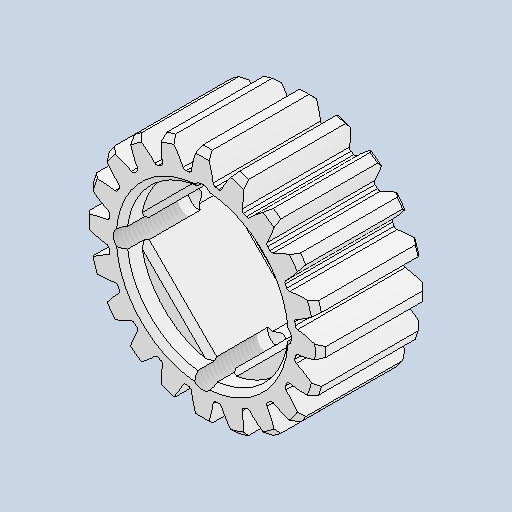
# Autodesk Inventor part: 스퍼 기어1
Saved by Autodesk Inventor 2025.3 (Build 293356030, 356C)
## iProperties
Created: 2025-10-17
Part Number: 스퍼 기어1
Material: PLA filament
Document SubType Name: Modeling
Designer: MSI
Categories: <?xml version="1.0" encoding="UTF-16"?> <MemberInstance><Categories><FamilyTemplate><FamilyTemplateParameter ValueType="xs:double" Id="1" ObjectReferenceKey="da_z" ObjectType="kUserParameterObject"/><FamilyTemplateParameter ValueType="xs:double" Id="2" ObjectReferenceKey="da_b" ObjectType="kUserParameterObject"/><FamilyTemplateParameter ValueType="xs:double" Id="3" ObjectReferenceKey="da_beta" ObjectType="kUserParameterObject"/><FamilyTemplateParameter ValueType="xs:double" Id="4" ObjectReferenceKey="da_da" ObjectType="kUserParameterObject"/><FamilyTemplateParameter ValueType="xs:double" Id="5" ObjectReferenceKey="da_aw" ObjectType="kUserParameterObject"/><FamilyTemplateParameter ValueType="xs:string" Id="6" ObjectReferenceKey="EAIAABAAAACIAQAAAAAAAIAAAAAAAAAA" ObjectType="83910656" SubObjectId="SurfaceGeometry"/></FamilyTemplate><ParamToTemplateMap><ParamToTemplate CategoryParameter="//CategoryParameter[@InternalName='046C89C9-8512-4d59-83FE-43B91F4F132A']" TemplateParameter="1"/><ParamToTemplate CategoryParameter="//CategoryParameter[@InternalName='2552DF32-E462-4b46-AEBF-C6C7768E72AC']" TemplateParameter="2"/><ParamToTemplate CategoryParameter="//CategoryParameter[@InternalName='C9EE641D-15FC-4fae-A226-E94C4372FDD7']" TemplateParameter="3"/><ParamToTemplate><ParamToTemplate CategoryParameter="//CategoryParameter[@InternalName='00B6519A-459B-49c7-AD84-2E56D39A5744']" ConstantValue="0.000000"/></ParamToTemplate><ParamToTemplate><ParamToTemplate CategoryParameter="//CategoryParameter[@InternalName='04B31F0E-C7A6-4894-AA32-9629BEFACF47']" ConstantValue="1.000000"/></ParamToTemplate><ParamToTemplate><ParamToTemplate CategoryParameter="//CategoryParameter[@InternalName='43CBEC2E-7847-49e7-A936-2F7889FCB2D9']" ConstantValue="0.250000"/></ParamToTemplate><ParamToTemplate><ParamToTemplate CategoryParameter="//CategoryParameter[@InternalName='B1EFC894-105D-4ebd-86BF-FA20ED196853']" ConstantValue="0.350000"/></ParamToTemplate><ParamToTemplate><ParamToTemplate CategoryParameter="//CategoryParameter[@InternalName='51175063-3D10-4879-93E8-6246FE8B403D']" ConstantValue="2060000000.000000"/></ParamToTemplate><ParamToTemplate><ParamToTemplate CategoryParameter="//CategoryParameter[@InternalName='A3A52E27-4454-46a9-B0BD-C932399B70AF']" ConstantValue="0.300000"/></ParamToTemplate><ParamToTemplate><ParamToTemplate CategoryParameter="//CategoryParameter[@InternalName='91B76062-C214-41d9-B1B9-14D2AB99603D']" ConstantValue="0.200000"/></ParamToTemplate><ParamToTemplate><ParamToTemplate CategoryParameter="//CategoryParameter[@InternalName='374E806E-8B8A-4dda-A9AA-1039D6500AD2']" ConstantValue="5.000000"/></ParamToTemplate><ParamToTemplate><ParamToTemplate CategoryParameter="//CategoryParameter[@InternalName='2D373A89-B862-43d6-8D0B-0CBF12AB9F6C']" ConstantValue="0.349066"/></ParamToTemplate><ParamToTemplate CategoryParameter="//CategoryParameter[@InternalName='37777632-D6A2-4fac-9D53-DB8ACD95C989']" TemplateParameter="4"/><ParamToTemplate CategoryParameter="//CategoryParameter[@InternalName='FD1017F1-B727-4f7e-9707-0F86F1FF9423']" TemplateParameter="5"/><ParamToTemplate><ParamToTemplate CategoryParameter="//CategoryParameter[@InternalName='9E1B4470-B2D3-4ff1-B813-535BB4CDF51A']" ConstantValue="3520000.000000"/></ParamToTemplate><ParamToTemplate><ParamToTemplate CategoryParameter="//CategoryParameter[@InternalName='F8452263-BFF6-458c-9FB1-07C4B99E95CD']" ConstantValue="11400000.000000"/></ParamToTemplate><ParamToTemplate><ParamToTemplate CategoryParameter="//CategoryParameter[@InternalName='3E3BB259-FD49-497f-8171-6EBC954A3479']" ConstantValue="2.000000"/></ParamToTemplate><ParamToTemplate CategoryParameter="//CategoryParameter[@InternalName='27C3BAF2-7550-4e4b-AE2C-0DB134B7D9B7']" TemplateParameter="6"/></ParamToTemplateMap><Category DisplayName="Gear" InternalName="DC85795E-93AB-48d5-8EEE-5A27447B64BD" Mnemonic="Gear"><CategoryParameter DisplayName="z" InternalName="046C89C9-8512-4d59-83FE-43B91F4F132A" Mnemonic="z"/><CategoryParameter DisplayName="b" InternalName="2552DF32-E462-4b46-AEBF-C6C7768E72AC" Mnemonic="b"/><CategoryParameter DisplayName="||b|" InternalName="C9EE641D-15FC-4fae-A226-E94C4372FDD7" Mnemonic="beta"/><CategoryParameter DisplayName="x" InternalName="00B6519A-459B-49c7-AD84-2E56D39A5744" Mnemonic="x"/><CategoryParameter DisplayName="a*" InternalName="04B31F0E-C7A6-4894-AA32-9629BEFACF47" Mnemonic="a"/><CategoryParameter DisplayName="c*" InternalName="43CBEC2E-7847-49e7-A936-2F7889FCB2D9" Mnemonic="c"/><CategoryParameter DisplayName="r|.f|*" InternalName="B1EFC894-105D-4ebd-86BF-FA20ED196853" Mnemonic="rf"/><CategoryParameter DisplayName="E" InternalName="51175063-3D10-4879-93E8-6246FE8B403D" Mnemonic="E"/><CategoryParameter DisplayName="||m|" InternalName="A3A52E27-4454-46a9-B0BD-C932399B70AF" Mnemonic="mi"/><Category DisplayName="SpurGear" InternalName="26C5A22E-A91E-4dfd-A3B3-23CCAFAE1764" Mnemonic="SpurGear"><CategoryParameter DisplayName="m" InternalName="91B76062-C214-41d9-B1B9-14D2AB99603D" Mnemonic="m"/><CategoryParameter DisplayName="P" InternalName="374E806E-8B8A-4dda-A9AA-1039D6500AD2" Mnemonic="PP"/><CategoryParameter DisplayName="||a|" InternalName="2D373A89-B862-43d6-8D0B-0CBF12AB9F6C" Mnemonic="alpha"/><CategoryParameter DisplayName="d|.a|" InternalName="37777632-D6A2-4fac-9D53-DB8ACD95C989" Mnemonic="da"/><CategoryParameter DisplayName="a|.w|" InternalName="FD1017F1-B727-4f7e-9707-0F86F1FF9423" Mnemonic="aw"/><CategoryParameter DisplayName="||s||.Flim|" InternalName="9E1B4470-B2D3-4ff1-B813-535BB4CDF51A" Mnemonic="sFlim"/><CategoryParameter DisplayName="||s||.Hlim|" InternalName="F8452263-BFF6-458c-9FB1-07C4B99E95CD" Mnemonic="sHlim"/><CategoryParameter DisplayName="유형" InternalName="3E3BB259-FD49-497f-8171-6EBC954A3479" Mnemonic="type"/><CategoryParameter DisplayName="PitchDiameter" InternalName="27C3BAF2-7550-4e4b-AE2C-0DB134B7D9B7" Mnemonic="IDS_PITCHDIAM"/></Category></Category></Categories></MemberInstance>
Density: 1.2 g/cm^3
Appearance: 일반
Mass: 16.1847 g
Surface Area: 81.0229 cm^2
Volume: 13.4873 cm^3
Author: MSI
Autodesk Inventor part; units mm, degrees
sketch "Sketch1" plane through (0, 0, 0) normal (0, 0, 1) x (1, 0, 0)
  circle A0 centre (0, 0) radius 22
  dimension "d0" = 44
  constraints: 1 centre point
  measures "d0" diameter of A0
extrude "Extrusion1" add sketch "Sketch1" along normal blind 20
chamfer "모따기1" distance 1 angle 45 2 edges at (-22, 0, 0) (-22, 0, 20)
ref_plane "Work Plane2" through (0, 0, 10) normal (0, 0, 1) x (1, 0, 0)
sketch "Sketch2" plane through (0, 0, 0) normal (0, 0, -1) x (-1, 0, 0)
  circle A0 centre (0, 0) radius 22 projected
  circle A1 centre (0, 0) radius 20
  dimension "d3" = 40
  constraints: 1 centre point, 1 coincident
  measures "d3" diameter of A1
surface extrude "피치 지름" sketch "Sketch2" against normal through all shown no curves A1
ref_plane "Work Plane8" through (0, 0, 0) normal (0.9876883, 0.1564345, 0) x (0, 0, 1)
ref_plane "Work Plane9" through (0, 0, 0) normal (1, 0, 0) x (0, 1, 0)
spur gear teeth "스퍼 기어" teeth 20 pitch diameter 40 tip diameter 44 root diameter 35 face width 20 start plane through (0, 0, 0) normal (0, 0, -1) x (-1, 0, 0)
fillet "모깎기1" radius 0.5 2 edges at (2.0569, 17.3787, 10) (3.4141, 17.1637, 10)
pattern_circular "원형 패턴1" count 20 over 360 about axis through (0, 0, 0) along (0, 0, 1) of "모깎기1"
sketch "스케치3" plane through (0, 0, 20) normal (0, 0, 1) x (1, 0, 0)
  point P0 (0, 0)
hole "구멍1" at (0, 0, 20) direction (0, 0, -1) diameter 30 end through all
sketch "스케치5" plane through (0, 0, 0) normal (0, 0, 1) x (1, 0, 0)
  line L0 (0, -16.1927) -> (16.1927, 0)
  line L1 (16.1927, 0) -> (0, 16.1927)
  line L2 (0, 16.1927) -> (-16.1927, 0)
  line L3 (-16.1927, 0) -> (0, -16.1927)
  line L4 (0, -16.1927) -> (0, 16.1927) construction
  line L5 (16.1927, 0) -> (-16.1927, 0) construction
  circle A0 centre (0, 0) radius 15 projected
  point P0 (-14.9483, -1.2445)
  point P1 (-14.9483, 1.2445)
  point P2 (-1.2445, 14.9483)
  point P3 (1.2445, 14.9483)
  point P4 (1.2445, -14.9483)
  point P5 (-1.2445, -14.9483)
  point P6 (14.9483, 1.2445)
  point P7 (14.9483, -1.2445)
  dimension "d74" = 22.9
  dimension "d75" = 22.9
  constraints: 12 end point, 2 midpoint, 2 parallel, 1 perpendicular, 1 vertical
  measures "d74" distance of L0.end L1.end
  measures "d75" distance of L0.start L0.end
extrude "돌출2" add sketch "스케치5" along normal blind 16.5 contours L3 A0 L0 | L0 A0 | A0 L3 | A0 L1 L0 | L3 L2 A0 | A0 L2 | L1 A0 | L2 L1 A0
chamfer "모따기2" distance 1 angle 45 10 edges at (0, 15, 20) (-15, 0, 0) (0.6228, -14.9871, 0) (-0.6228, -14.9871, 0) (15, 0, 0) (0, 15, 0) (-8.0964, 8.0964, 0) (8.0964, 8.0964, 0) (8.0964, -8.0964, 0) (-8.0964, -8.0964, 0)
sketch "스케치6" plane through (0, 0, 20) normal (0, 0, -1) x (-1, 0, 0)
  line L0 (0, 0) -> (-14.75, 0) construction
  dimension "d78" = 14.75
  constraints: 2 end point, 1 coincident, 1 horizontal
  measures "d78" distance of L0.start L0.end
hole "구멍3" at (14.75, 0, 20) direction (0, 0, -1) diameter 3.6881 depth 14 tip angle 118 thread size "M4.5x0.75" class "6H" standard "ISO Metric profile"
pattern_circular "원형 패턴2" count 4 over 360 about axis through (0, 0, -45.3615) along (0, 0, 1) of "구멍3"
chamfer "모따기3" distance 1 angle 45 4 edges at (-8.0964, -8.0964, 16.5) (-8.0964, 8.0964, 16.5) (8.0964, 8.0964, 16.5) (8.0964, -8.0964, 16.5)
equation "\"d0\" = da_da"
equation "\"d1\" = da_b"
equation "\"d75\" = d74"
equation "\"d3\" = da_d"
equation "\"joint4_belt_centor\" = 157.367"
equation "\"joint4_axis2_L\" = 58.803"
equation "\"joint4_axis2_b1\" = 35"
equation "\"joint4_axis2_d\" = 19"
equation "\"joint4_miter_m\" = 2"
equation "\"joint4_miter_a\" = 20deg"
equation "\"joint4_miter_z\" = 79"
equation "\"joint4_miter_b\" = 6.90139"
equation "\"joint4_axis3_L\" = 23.5"
equation "\"joint3_belt_centor\" = 157.367"
equation "\"joint3_axis2_L\" = 63.75"
equation "\"joint3_axis2_b1\" = 38"
equation "\"joint3_axis2_d\" = 29"
equation "\"joint3_planetary_m\" = 2"
equation "\"joint3_planetary_a\" = 20deg"
equation "\"joint3_planetary_np\" = 4"
equation "\"joint3_sun_b\" = 19"
equation "\"joint3_planet_b\" = 19"
equation "\"joint3_ring_b\" = 18"
equation "\"joint3_axis3_d\" = 29"
equation "\"joint3_miter_m\" = 4"
equation "\"joint3_miter_a\" = 20deg"
equation "\"joint3_miter_z1\" = 26"
equation "\"joint3_miter_z2\" = 39"
equation "\"joint3_miter_b\" = 25.07657"
equation "\"joint3_axis4_L\" = 43.706"
equation "\"da_da\" = 44"
equation "\"da_b\" = 20"
equation "\"da_d\" = 40"
body "Solid1"
body "Srf1"
